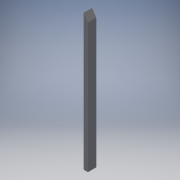
# Autodesk Inventor part: R long Angle
Saved by Autodesk Inventor 2018.2 (Build 222227000, 227)
## iProperties
Created: 2018-01-29
Part Number: R long Angle
Material: Generic
Document SubType Name: Modeling
Designer: Orangeracer
Density: 1 g/cm^3
Appearance: Default
Author: Orangeracer
Autodesk Inventor part; units mm, degrees
ref_plane "YZ Plane" through (0, 0, 0) normal (1, 0, 0) x (0, 1, 0)
ref_plane "XZ Plane" through (0, 0, 0) normal (0, 1, 0) x (-1, 0, 0)
ref_plane "XY Plane" through (0, 0, 0) normal (0, 0, 1) x (1, 0, 0)
sketch "Sketch1" plane through (0, 0, 0) normal (0, 0, 1) x (1, 0, 0)
  line L0 (0, 0) -> (-50.8, 0)
  line L1 (-50.8, 0) -> (-50.8, 25.4)
  line L2 (0, 0) -> (-50.8, 25.4)
  line L3 (-50.8, 0) -> (0, 0)
  line L4 (0, 0) -> (0, -571.5)
  line L5 (0, -571.5) -> (-50.8, -571.5)
  line L6 (-50.8, -571.5) -> (-50.8, 0)
  dimension "d1" = 25.4
  dimension "d2" = 50.8
  dimension "d3" = 25.4
  dimension "d4" = 571.5
  dimension "d5" = 50.8
  constraints: 14 end point, 2 horizontal, 2 parallel, 2 perpendicular
  measures "d1" distance of L0.end L1.end
  measures "d2" distance of L0.start L0.end
  measures "d3" vertical distance of L0.start L1.end
  measures "d4" distance of L5.end L0.end
  measures "d5" distance of L4.end L5.end
extrude "Extrusion1" add sketch "Sketch1" along normal blind 25.4
body "Solid1"
